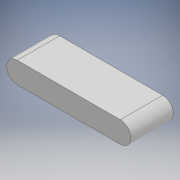
# Autodesk Inventor part: C-PAN
Saved by Autodesk Inventor 2018 (Build 220112000, 112)
## iProperties
Created: 2018-01-22
Part Number: C-PAN
Material: Generic
Document SubType Name: Modeling
Designer: gevon
Density: 1 g/cm^3
Appearance: Default
Author: gevon
Autodesk Inventor part; units mm, degrees
ref_plane "YZ Plane" through (0, 0, 0) normal (1, 0, 0) x (0, 1, 0)
ref_plane "XZ Plane" through (0, 0, 0) normal (0, 1, 0) x (-1, 0, 0)
ref_plane "XY Plane" through (0, 0, 0) normal (0, 0, 1) x (1, 0, 0)
sketch "Sketch1" plane through (0, 0, 0) normal (0, 1, 0) x (-1, 0, 0)
  arc A0 (-93.5462, 17.5) -> (-93.5462, -17.5) centre (-93.5462, 0) ccw
  arc A1 (-93.5462, 17.5) -> (-93.5462, -17.5) centre (-93.5462, 0) ccw
  line L0 (-68.5462, -17.5) -> (51.4538, -17.5)
  line L1 (51.4538, -17.5) -> (51.4538, 12.6842)
  line L2 (51.4538, 12.6842) -> (-68.5462, 12.6842)
  line L3 (-68.5462, 12.6842) -> (-68.5462, -17.5)
  line L4 (-68.5462, -17.5) -> (-93.5462, -17.5)
  arc A2 (76.4538, -17.5) -> (76.4538, 17.5) centre (76.4538, 0) ccw
  line L5 (51.4538, -17.5) -> (76.4538, -17.5)
  line L6 (76.4538, 17.5) -> (-93.5462, 17.5)
  point P0 (0, 0)
  dimension "d0" = 35
  dimension "d1" = 120
  dimension "d2" = 25
  dimension "d3" = 35
  dimension "d4" = 25
  constraints: 14 end point, 6 point on circle, 3 centre point, 3 parallel, 2 horizontal, 1 coincident, 1 concentric, 1 perpendicular, 1 tangent
  measures "d0" diameter of A0
  measures "d1" distance of L2.end L1.end
  measures "d2" distance from line of A0.centre L3
  measures "d3" diameter of A2
  measures "d4" distance from line of L1 A2.centre
extrude "Extrusion1" add sketch "Sketch1" along normal blind 65 contours L6 A2 L5 L1 L2 L3 L4 A0
sketch "Sketch2" plane through (0, 65, 0) normal (0, 1, 0) x (1, 0, 0)
  arc A0 (-69.3673, -11.4905) -> (-75.5737, -13.4713) centre (-76.4538, 0) ccw
  arc A1 (92.6661, -13.4713) -> (86.972, -11.7911) centre (93.5462, 0) ccw
  line L0 (-51.4538, -12.6842) -> (-51.4538, 17.5) projected
  line L1 (68.5462, 17.5) -> (68.5462, -12.6842) projected
  line L2 (93.5462, -13.5) -> (68.5462, -12.6842)
  line L3 (-76.4538, -13.5) -> (-51.4538, -12.6842)
  line L4 (68.5462, -11.1899) -> (86.972, -11.7911)
  line L5 (-51.4538, -11.8536) -> (-69.3673, -11.4905)
  line L6 (-51.4538, -11.8536) -> (-51.4267, -12.6833)
  line L7 (68.5462, -11.1899) -> (68.5462, -12.6842)
  point P0 (0, 0)
  dimension "d7" = 27
  dimension "d8" = 27
  dimension "d9" = 25
  dimension "d10" = 25
  constraints: 12 end point, 6 point on circle, 5 point on line, 2 centre point, 1 collinear, 1 parallel, 1 perpendicular
  measures "d7" diameter of A0
  measures "d8" diameter of A1
  measures "d9" distance from line of L0 A0.centre
  measures "d10" distance from line of L1 A1.centre
extrude "Extrusion2" cut sketch "Sketch2" against normal blind 65 contours L5 L0 L3 A0 | L2 L1 L4 A1
sketch "Sketch4" plane through (0, 0, 0) normal (0, -1, 0) x (1, 0, 0)
  arc A0 (-76.4538, 13.5) -> (-69.3673, 11.4905) centre (-76.4538, 0) ccw projected
  arc A1 (-76.4538, 17.5) -> (-76.4538, -17.5) centre (-76.4538, 0) ccw
  arc A2 (93.5462, -17.5) -> (93.5462, 17.5) centre (93.5462, 0) ccw projected
  arc A3 (93.5462, -17.5) -> (93.5462, 17.5) centre (93.5462, 0) ccw
  line L0 (-76.4538, 17.5) -> (93.5462, 17.5) projected
  line L1 (-76.4538, 17.5) -> (93.5462, 17.5)
  line L2 (-51.4538, -17.5) -> (-76.4538, -17.5) projected
  line L3 (-76.4538, -17.5) -> (93.5462, -17.5)
  point P0 (0, 0)
  constraints: 4 end point, 4 point on circle, 2 centre point, 2 coincident, 2 collinear, 1 tangent
extrude "Extrusion4" add sketch "Sketch4" along normal blind 5
sketch "Sketch5" plane through (0, 0, 0) normal (0, 1, 0) x (1, 0, 0)
  line L0 (-69.3673, -11.4905) -> (-51.4538, -11.8536) projected
  line L1 (68.5462, 17.5) -> (68.5462, -11.1899) projected
  line L2 (-51.4538, -11.8536) -> (68.5462, -11.8536)
  line L3 (68.5462, -11.8536) -> (68.5462, -8.8458)
  line L4 (68.5462, -8.8458) -> (-51.4538, -8.8458)
  line L5 (-51.4538, -8.8458) -> (-51.4538, -11.8536)
  point P0 (0, 0)
  constraints: 8 end point, 2 parallel, 1 horizontal, 1 perpendicular, 1 point on line
extrude "Extrusion5" add sketch "Sketch5" along normal blind 2
sketch "Sketch6" plane through (68.5462, 0, 8.8458) normal (0, 0, -1) x (-1, 0, 0)
  point P0 (68.5462, 0)
sketch "Sketch7" plane through (0, 0, 0) normal (0, 1, 0) x (1, 0, 0)
  line L0 (68.5462, -11.8536) -> (68.5462, -11.1899) projected
  line L1 (68.5462, -11.1899) -> (86.972, -11.7911) projected
  line L2 (68.5462, -11.8536) -> (86.972, -11.7911)
  line L3 (68.5462, -8.8458) -> (68.5462, -11.1899) projected
  line L4 (86.972, -11.7911) -> (68.5462, -11.1899)
  line L5 (68.5462, -11.1899) -> (68.5266, -11.7911)
  point P0 (0, 0)
  constraints: 6 end point, 1 perpendicular
extrude "Extrusion6" add sketch "Sketch7" along normal blind 65
sketch "Sketch8" plane through (-51.4538, 65, 11.8536) normal (1, 0, 0) x (0, 0, -1)
  line L0 (0, 0) -> (29.3536, 0) projected
  line L1 (0, 0) -> (4.0071, 0)
  line L2 (4.0071, 0) -> (4.0071, -2.0911)
  line L3 (4.0071, -2.0911) -> (0, -2.0911)
  line L4 (0, -2.0911) -> (0, 0)
  point P0 (11.8536, -65)
  constraints: 8 end point, 2 parallel, 1 horizontal, 1 perpendicular
extrude "Extrusion7" add sketch "Sketch8" along normal blind 120
fillet "Fillet1" radius 0.5 1 edges at (-69.3673, 32.5, 11.4905)
fillet "Fillet2" radius 0.5 1 edges at (86.972, 32.5, 11.7911)
chamfer "Chamfer1" distance 1 angle 45 1 edges at (8.5462, 2, 8.8458)
chamfer "Chamfer2" distance 1 angle 45 1 edges at (8.5462, 62.9089, 7.8466)
sketch "Sketch9" plane through (0, 0, 0) normal (0, 1, 0) x (1, 0, 0)
  arc A0 (93.5462, -17.5) -> (93.5462, 17.5) centre (93.5462, 0) ccw projected
  line L0 (93.5462, 17.5) -> (68.5462, 17.5) projected
  line L1 (93.5462, 17.5) -> (93.5462, 17.5)
  circle A1 centre (93.5462, 0) radius 2
  line L2 (-76.4538, 17.5) -> (93.5462, 17.5) projected
  line L3 (-76.4538, -17.5) -> (93.5462, -17.5) projected
  circle A2 centre (-76.4538, 0) radius 2
  point P0 (0, 0)
  dimension "d39" = 4
  dimension "d40" = 4
  constraints: 2 centre point, 2 end point, 1 coincident, 1 perpendicular
  measures "d39" diameter of A1
  measures "d40" diameter of A2
extrude "Extrusion8" add sketch "Sketch9" along normal blind 5
fillet "Fillet3" radius 0.5 2 edges at (91.5462, 5, 0) (-78.4538, 5, 0)
sketch "Sketch10" plane through (-51.4538, 65, -17.5) normal (0, 0, -1) x (-1, 0, 0)
  circle A0 centre (-125, -5) radius 1.75
  circle A1 centre (-125, -60) radius 1.75
  line L0 (25, -70) -> (-145, -70) projected
  line L1 (-120, -65) -> (-120, 0) projected
  line L2 (-145, 0) -> (-120, 0) projected
  circle A2 centre (5, -60) radius 1.75
  circle A3 centre (5, -5) radius 1.75
  line L3 (0, -65) -> (0, 0) projected
  line L4 (0, 0) -> (25, 0) projected
  point P0 (-51.4538, -65)
  dimension "d44" = 3.5
  dimension "d45" = 3.5
  dimension "d46" = 10
  dimension "d47" = 5
  dimension "d48" = 5
  dimension "d49" = 3.5
  dimension "d50" = 3.5
  dimension "d51" = 5
  dimension "d52" = 5
  dimension "d53" = 5
  dimension "d54" = 10
  constraints: 4 centre point
  measures "d44" diameter of A0
  measures "d45" diameter of A1
  measures "d46" distance from line of A1.centre L0
  measures "d47" distance from line of L1 A1.centre
  measures "d48" distance from line of L2 A0.centre
  measures "d49" diameter of A2
  measures "d50" diameter of A3
  measures "d51" distance from line of L3 A3.centre
  measures "d52" distance from line of L4 A3.centre
  measures "d53" distance from line of L3 A2.centre
  measures "d54" distance from line of L0 A2.centre
extrude "Extrusion9" cut sketch "Sketch10" against normal blind 10
sketch "Sketch11" plane through (0, 65, 0) normal (0, 1, 0) x (1, 0, 0)
  point P0 (0, 0)
sketch "Sketch12" plane through (0, 65, 0) normal (0, 1, 0) x (1, 0, 0)
  circle A0 centre (73.5462, -2.5) radius 2
  circle A1 centre (-56.4538, -2.5) radius 2
  line L0 (68.5462, 17.5) -> (68.5462, -7.8466) projected
  line L1 (93.5462, 17.5) -> (68.5462, 17.5) projected
  line L2 (-51.4538, -7.8466) -> (-51.4538, 17.5) projected
  arc A2 (93.5462, -17.5) -> (93.5462, 17.5) centre (93.5462, 0) ccw projected
  point P0 (0, 0)
  dimension "d57" = 4
  dimension "d58" = 4
  dimension "d59" = 5
  dimension "d60" = 20
  dimension "d61" = 5
  dimension "d62" = 20
  constraints: 2 centre point
  measures "d57" diameter of A0
  measures "d58" diameter of A1
  measures "d59" distance from line of L0 A0.centre
  measures "d60" distance from line of L1 A0.centre
  measures "d61" distance from line of L2 A1.centre
  measures "d62" horizontal distance of A2.centre A0.centre
extrude "Extrusion10" cut sketch "Sketch12" against normal blind 10
body "Solid1"
